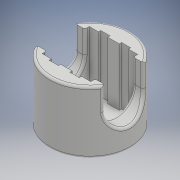
# Autodesk Inventor part: Soporte Ultrasonicos Maxsonar
Saved by Autodesk Inventor 2019 (Build 230136000, 136)
## iProperties
Created: 2018-04-27
Part Number: Soporte Ultrasonicos Maxsonar
Material: Generic
Document SubType Name: Modeling
Designer: lim14373
Density: 1 g/cm^3
Appearance: Default
Author: lim14373
Autodesk Inventor part; units mm, degrees
ref_plane "YZ Plane" through (0, 0, 0) normal (1, 0, 0) x (0, 1, 0)
ref_plane "XZ Plane" through (0, 0, 0) normal (0, 1, 0) x (-1, 0, 0)
sketch "Sketch1" plane through (0, 0, 0) normal (0, 0, 1) x (1, 0, 0)
  line L0 (-12.5, 24.4) -> (12.5, 24.4)
  line L1 (12.5, 24.4) -> (12.5, 0)
  line L2 (12.5, 0) -> (-12.5, 0)
  line L3 (-12.5, 0) -> (-12.5, 24.4)
  point P0 (0, 0)
  point P1 (0, 0)
  dimension "d0" = 25
  dimension "d1" = 24.4
  constraints: 8 end point, 2 horizontal, 2 vertical, 1 coincident, 1 midpoint
  measures "d0" distance of L0.start L0.end
  measures "d1" distance of L0.end L1.end
extrude "Extrusion1" add sketch "Sketch1" along normal blind 2
ref_plane "Work Plane1" through (0, 0, 22.86) normal (0, 0, 1) x (1, 0, 0)
sketch "Sketch4" plane through (0, 0, 0) normal (0, 0, -1) x (-1, 0, 0)
  arc A0 (1.85, 10.0982) -> (-1.85, 10.0982) centre (0, 12.2) ccw
  arc A1 (-1.85, 5.4) -> (1.85, 5.4) centre (0, 5.4) ccw
  line L0 (1.85, 10.0982) -> (1.85, 5.4)
  line L1 (-1.85, 10.0982) -> (-1.85, 5.4)
  line L2 (12.5, 0) -> (12.5, 24.4) projected
  line L3 (12.5, 24.4) -> (-12.5, 24.4) projected
  point P0 (0, 0)
  point P1 (12.5, 12.2)
  point P2 (0, 24.4)
  dimension "d20" = 3.7
  dimension "d21" = 11.45
  dimension "d22" = 2.8
  constraints: 4 end point, 4 point on circle, 2 centre point, 2 horizontal alignment, 2 midpoint, 2 tangent, 2 vertical, 1 vertical alignment
  measures "d20" distance between parallel lines of L0 L1
  measures "d22" radius of A0
extrude "Extrusion4" cut sketch "Sketch4" against normal blind 1
sketch "Sketch5" plane through (0, 0, 1) normal (0, 0, -1) x (-1, 0, 0)
  circle A0 centre (0, 5.4) radius 0.75
  circle A1 centre (0, 12.2) radius 0.75
  arc A2 (1.85, 10.0982) -> (-1.85, 10.0982) centre (0, 12.2) ccw projected
  arc A3 (-1.85, 5.4) -> (1.85, 5.4) centre (0, 5.4) ccw projected
  point P0 (0, 0)
  dimension "d25" = 1.5
  constraints: 2 centre point, 2 concentric, 1 equal radius
  measures "d25" diameter of A1
extrude "Extrusion5" cut sketch "Sketch5" against normal through all
sketch "Sketch6" plane through (0, 0, 0) normal (0, 0, -1) x (-1, 0, 0)
  line L0 (-10.5, 22.45) -> (-7.5, 22.45)
  line L1 (-7.5, 22.45) -> (-7.5, 1.95)
  line L2 (-7.5, 1.95) -> (-10.5, 1.95)
  line L3 (-10.5, 1.95) -> (-10.5, 22.45)
  line L4 (7.5, 22.45) -> (10.5, 22.45)
  line L5 (10.5, 22.45) -> (10.5, 1.95)
  line L6 (10.5, 1.95) -> (7.5, 1.95)
  line L7 (7.5, 1.95) -> (7.5, 22.45)
  line L8 (12.5, 24.4) -> (-12.5, 24.4) projected
  line L9 (-12.5, 0) -> (12.5, 0) projected
  circle A0 centre (0, 12.2) radius 0.75 projected
  point P0 (0, 0)
  point P1 (-7.5, 12.2)
  dimension "d30" = 3
  dimension "d31" = 3
  dimension "d32" = 7.5
  dimension "d33" = 7.5
  dimension "d47" = 20.5
  constraints: 16 end point, 4 horizontal, 4 vertical, 3 horizontal alignment, 1 midpoint, 1 point on line
  measures "d30" distance of L0.start L0.end
  measures "d31" distance of L4.start L4.end
  measures "d32" distance from line of A0.centre L7
  measures "d33" distance from line of L1 A0.centre
  measures "d47" distance of L2.end L0.start
extrude "Extrusion6" cut sketch "Sketch6" against normal through all contours L0 L1 L2 L3 | L4 L5 L6 L7
sketch "Sketch9" plane through (0, 0, 2) normal (0, 0, 1) x (1, 0, 0)
  line L0 (-12.5, 0) -> (12.5, 0)
  line L1 (12.5, 0) -> (12.5, 2)
  line L2 (12.5, 2) -> (-12.5, 2)
  line L3 (-12.5, 2) -> (-12.5, 0)
  line L4 (-12.5, 22.4) -> (12.5, 22.4)
  line L5 (12.5, 22.4) -> (12.5, 24.4)
  line L6 (12.5, 24.4) -> (-12.5, 24.4)
  line L7 (-12.5, 24.4) -> (-12.5, 22.4)
  line L8 (10.5, 0) -> (12.5, 0)
  line L9 (12.5, 0) -> (12.5, 24.4)
  line L10 (12.5, 24.4) -> (10.5, 24.4)
  line L11 (10.5, 24.4) -> (10.5, 0)
  line L12 (-10.5, 0) -> (-12.5, 0)
  line L13 (-12.5, 0) -> (-12.5, 24.4)
  line L14 (-12.5, 24.4) -> (-10.5, 24.4)
  line L15 (-10.5, 24.4) -> (-10.5, 0)
  point P0 (0, 0)
  dimension "d48" = 2
  dimension "d49" = 2
  dimension "d50" = 2
  dimension "d51" = 2
  constraints: 32 end point, 8 horizontal, 8 vertical, 2 coincident
  measures "d48" distance of L6.end L14.end
  measures "d49" distance of L5.end L10.end
  measures "d50" distance between parallel lines of L6 L4
  measures "d51" distance between parallel lines of L0 L2
extrude "Extrusion9" add sketch "Sketch9" along normal blind 25 contours L3 L2 L15 L0 | L15 L2 L11 L0 | L13 L4 L15 L2 | L11 L2 L1 L0 | L7 L6 L15 L4 | L11 L4 L9 L2 | L15 L6 L11 L4 | L11 L6 L5 L4
sketch "Sketch11" plane through (12.5, 0, 0) normal (1, 0, 0) x (0, 0, -1)
  arc A0 (-17, 3.95) -> (-17, 20.45) centre (-17, 12.2) ccw
  line L0 (-17, 3.95) -> (-27, 3.95)
  line L1 (-27, 3.95) -> (-27, 20.45)
  line L2 (-27, 20.45) -> (-17, 20.45)
  line L3 (-27, 0) -> (-27, 24.4) projected
  point P0 (0, 0)
  point P1 (-27, 12.2)
  dimension "d54" = 16.5
  dimension "d56" = 10
  constraints: 6 end point, 2 horizontal, 2 point on circle, 2 tangent, 1 centre point, 1 horizontal alignment, 1 midpoint, 1 point on line, 1 vertical
  measures "d54" distance of L0.end L1.end
  measures "d56" distance from line of A0.centre L1
extrude "Extrusion10" cut sketch "Sketch11" against normal through all
sketch "Sketch12" plane through (0, 0, 27) normal (0, 0, 1) x (1, 0, 0)
  line L0 (-6.5, 1) -> (-2.5, 1)
  line L1 (-2.5, 1) -> (-2.5, 2)
  line L2 (-2.5, 2) -> (-6.5, 2)
  line L3 (-6.5, 2) -> (-6.5, 1)
  line L4 (2.5, 1) -> (6.5, 1)
  line L5 (6.5, 1) -> (6.5, 2)
  line L6 (6.5, 2) -> (2.5, 2)
  line L7 (2.5, 2) -> (2.5, 1)
  line L8 (-6.5, 22.4) -> (-2.5, 22.4)
  line L9 (-2.5, 22.4) -> (-2.5, 23.4)
  line L10 (-2.5, 23.4) -> (-6.5, 23.4)
  line L11 (-6.5, 23.4) -> (-6.5, 22.4)
  line L12 (2.5, 22.4) -> (6.5, 22.4)
  line L13 (6.5, 22.4) -> (6.5, 23.4)
  line L14 (6.5, 23.4) -> (2.5, 23.4)
  line L15 (2.5, 23.4) -> (2.5, 22.4)
  line L16 (10.5, 2) -> (-10.5, 2) projected
  line L17 (-10.5, 22.4) -> (10.5, 22.4) projected
  line L18 (10.5, 22.4) -> (10.5, 20.45) projected
  line L19 (-10.5, 20.45) -> (-10.5, 22.4) projected
  point P0 (0, 0)
  dimension "d59" = 1
  dimension "d60" = 4
  dimension "d61" = 1
  dimension "d62" = 4
  dimension "d63" = 1
  dimension "d64" = 4
  dimension "d65" = 1
  dimension "d66" = 4
  dimension "d67" = 4
  dimension "d68" = 4
  constraints: 32 end point, 8 horizontal, 8 vertical, 4 point on line, 2 vertical alignment
  measures "d59" distance of L2.end L0.start
  measures "d60" distance of L1.end L2.end
  measures "d61" distance of L6.end L4.start
  measures "d62" distance of L5.end L6.end
  measures "d63" distance of L10.end L8.start
  measures "d64" distance of L9.end L10.end
  measures "d65" distance of L14.end L12.start
  measures "d66" distance of L13.end L14.end
  measures "d67" distance between parallel lines of L13 L18
  measures "d68" distance between parallel lines of L19 L11
extrude "Extrusion11" cut sketch "Sketch12" against normal blind 25
fillet "Fillet5" radius 1 2 edges at (-7.5, 12.2, 2) (7.5, 12.2, 2)
fillet "Fillet6" radius 1 2 edges at (7.5, 12.2, 0) (-7.5, 12.2, 0)
sketch "Sketch13" plane through (0, 0, 0) normal (0, 0, -1) x (-1, 0, 0)
  circle A0 centre (0, 12.2) radius 17.4668
  circle A1 centre (0, 12.2) radius 0.75 projected
  line L0 (-12.5, 0) -> (-12.5, 24.4)
  line L1 (-12.5, 0) -> (12.5, 0)
  line L2 (12.5, 0) -> (12.5, 24.4)
  line L3 (12.5, 24.4) -> (-12.5, 24.4)
  line L4 (-12.5, 24.4) -> (-12.5, 0)
  point P0 (0, 0)
  constraints: 10 end point, 2 parallel, 2 point on circle, 1 centre point, 1 concentric, 1 horizontal, 1 perpendicular
extrude "Extrusion12" add sketch "Sketch13" against normal up to surface (27 mm away) contours A0 L2 | L3 A0 | A0 L1 | L0 A0
extrude "Extrusion13" cut sketch "Sketch11" along normal through all both and the other way through all
fillet "Fillet9" radius 1 16 edges at (17.4668, 12.2395, 8.7501) (-17.4668, 12.2395, 8.7501) (15.3957, 20.45, 22) (-15.3957, 20.45, 22) (15.3957, 3.95, 22) (-15.3957, 3.95, 22) (-10.5, 3.95, 22) (-10.5, 20.45, 22) (-10.5, 12.2, 8.75) (10.5, 20.45, 22) (10.5, 3.95, 22) (10.5, 12.2, 8.75) (-14.087, 1.873, 27) (2.4489, -5.0943, 27) (0, 29.6668, 27) (12.5, 24.4, 0)
fillet "Fillet10" radius 1 6 edges at (10.5, 12.2, 0) (8.5, 1.95, 0) (8.5, 22.45, 0) (-10.5, 12.2, 0) (-8.5001, 22.45, 0) (-8.5001, 1.95, 0)
body "Solid1"
